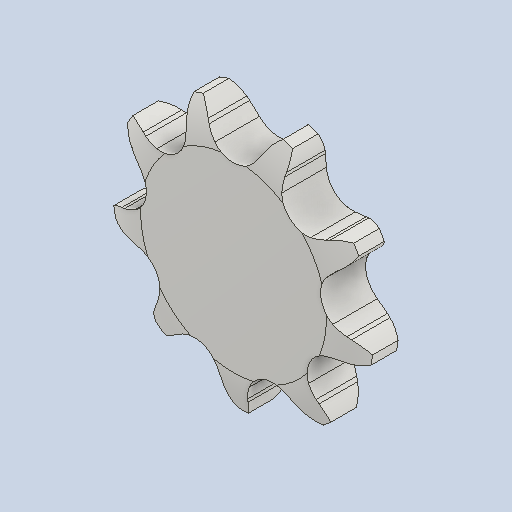
# Autodesk Inventor part: Rueda dentada de cadena de rodillos2
Saved by Autodesk Inventor 2022.1 (Build 261234000, 234)
## iProperties
CustomPartVersion: 1
Created: 2021-09-11
Part Number: Rueda dentada de cadena de rodillos2
Material: Steel
Document SubType Name: Modeling
Designer: seb_0
Density: 1 g/cm^3
Appearance: Steel
Author: seb_0
Autodesk Inventor part; units mm, degrees
ref_plane "YZ Plane" through (0, 0, 0) normal (1, 0, 0) x (0, 1, 0)
ref_plane "XZ Plane" through (0, 0, 0) normal (0, 1, 0) x (-1, 0, 0)
ref_plane "XY Plane" through (0, 0, 0) normal (0, 0, 1) x (1, 0, 0)
sketch "Perfil de diente teórico" plane through (0, 0, 0) normal (0, 0, 1) x (1, 0, 0)
  circle A0 centre (0, 0) radius 23.2077 construction
  line L0 (0, 0) -> (0, 23.2077) construction
  line L1 (0, 0) -> (14.9176, 17.7781) construction
  circle A1 centre (0, 0) radius 26.5706
  arc A2 (-3.8328, 19.7968) -> (3.8328, 19.7968) centre (0, 23.2077) ccw
  line L2 (0, 23.2077) -> (14.9176, 17.7781) construction
  line L3 (0, 23.2077) -> (6.0718, 28.6112) construction
  line L4 (6.0718, 28.6112) -> (-5.4235, 22.004) construction
  arc A3 (8.1227, 25.2986) -> (5.814, 22.6835) centre (13.3662, 18.3428) ccw
  arc A4 (-5.814, 22.6835) -> (-8.1227, 25.2986) centre (-13.3662, 18.3428) ccw
  line L5 (-13.3662, 18.3428) -> (-5.814, 22.6835) construction
  arc A5 (-5.4235, 22.004) -> (-3.8328, 19.7968) centre (6.0718, 28.6112) ccw
  line L6 (-5.4235, 22.004) -> (-5.814, 22.6835)
  arc A6 (3.8328, 19.7968) -> (5.4235, 22.004) centre (-6.0718, 28.6112) ccw
  line L7 (5.814, 22.6835) -> (5.4235, 22.004)
  line L8 (0, 0) -> (9.0877, 24.9682) construction
  point P0 (7.4588, 20.4929)
  dimension "d0" = 46.4154
  dimension "d2" = 40
  dimension "d3" = 5.1308
  dimension "d10" = 131.667
  dimension "d11" = 11.778
  dimension "d12" = 8.128
  dimension "d13" = 13.2588
  dimension "d14" = 14.224
  dimension "d23" = 4.7625
  constraints: 18 end point, 15 point on circle, 7 centre point, 3 coincident, 3 point on line, 3 symmetric about line, 3 tangent, 1 equal radius, 1 midpoint, 1 parallel, 1 vertical, 1 other
  measures "d0" diameter of A0
  measures "d2" angle of L1 L0
  measures "d3" radius of A2
  measures "d10" angle of L3 L0
  measures "d11" angle of L4 L3
  measures "d12" distance of L2.start L3.end
  measures "d13" distance of L3.end L4.end
  measures "d14" distance of A3.centre L0.end
  measures "d23" distance from line of L8.end L2
sketch "Perfil de diente" plane through (0, 0, 0) normal (0, 0, 1) x (1, 0, 0)
  arc A0 (-4.6501, 21.0393) -> (4.6501, 21.0393) centre (0, 23.2077) ccw
  arc A1 (7.8744, 25.377) -> (4.6501, 21.0393) centre (16.8048, 15.3715) ccw
  arc A2 (-4.6501, 21.0393) -> (-7.8744, 25.377) centre (-16.8048, 15.3715) ccw
  line L0 (0, 0) -> (0, 23.2077) construction
  line L1 (0, 23.2077) -> (4.6501, 21.0393) construction
  line L2 (0, 23.2077) -> (-4.6501, 21.0393) construction
  circle A3 centre (0, 0) radius 26.5706 projected
  dimension "d44" = 130
  dimension "d45" = 13.4112
  dimension "d46" = 5.1308
  constraints: 9 point on circle, 6 end point, 3 centre point, 2 tangent, 1 coincident, 1 equal radius, 1 vertical, 1 other
  measures "d44" angle of L2 L1
  measures "d45" radius of A1
  measures "d46" radius of A0
sketch "Perfil de sección" plane through (0, 0, 0) normal (1, 0, 0) x (0, 1, 0)
  line L0 (26.5706, 0) -> (-26.5706, 0) projected
  line L1 (9.7135, 4.5838) -> (-9.7135, 4.5838)
  line L2 (-9.7135, 4.5838) -> (-9.7135, -4.5838)
  line L3 (-9.7135, -4.5838) -> (9.7135, -4.5837)
  line L4 (9.7135, -4.5837) -> (9.7135, 4.5838)
  line L5 (9.7135, 4.5838) -> (26.5706, 4.5838) construction
  line L6 (26.5706, 4.5838) -> (26.5706, -4.5838) construction
  line L7 (26.5706, -4.5838) -> (9.7135, -4.5838) construction
  line L8 (9.7135, -4.5838) -> (9.7135, 4.5838)
  arc A0 (26.5706, 2.5994) -> (18.8852, 4.5838) centre (18.8852, -11.2913) ccw
  arc A1 (18.8852, -4.5838) -> (26.5706, -2.5994) centre (18.8852, 11.2913) ccw
  line L9 (18.8852, 4.5838) -> (0, 4.5838)
  line L10 (0, 4.5838) -> (0, -4.5838)
  line L11 (0, -4.5838) -> (18.8852, -4.5838)
  line L12 (0, 4.5838) -> (0, -4.5838)
  line L13 (26.5706, 2.5994) -> (26.5706, -2.5994)
  point P0 (0, 0)
  point P1 (0, 0)
  dimension "d30" = 9.1675
  dimension "d31" = 19.427
  dimension "d32" = 9.1675
  dimension "d33" = 1.9844
  dimension "d34" = 15.875
  dimension "d43" = 4.5838
  constraints: 26 end point, 7 midpoint, 5 perpendicular, 4 parallel, 4 point on circle, 3 point on line, 3 symmetric about line, 2 centre point, 2 horizontal, 2 tangent, 1 collinear, 1 other
  measures "d30" distance between parallel lines of L7 L5
  measures "d31" distance between parallel lines of L2 L4
  measures "d32" distance between parallel lines of L3 L1
  measures "d33" distance from line of L13.start L5
  measures "d34" radius of A0
  measures "d43" distance between parallel lines of L3 L0
revolve "Cubierta" add sketch "Perfil de sección" angle 360 about axis through (0, 0, 4.5838) along (0, 0, -1) contours L10 L3 L2 L0 | L0 L2 L1 L10
revolve "Ramal" add sketch "Perfil de sección" angle 360 about axis through (0, 0, 4.5838) along (0, 0, -1) contours L13 A1 L11 L4 L0 | L0 L4 L9 A0 L13 | L4 L3 L10 L0 | L0 L10 L1 L4
pattern_of_one "Patrón de ramal"
extrude "Diente teórico" cut sketch "Perfil de diente teórico" along normal through all both and the other way through all contours A3 L7 A6 A2 A5 L6 A4 A1 picked at (0.2056, 23.6569)
extrude "Diente" [suppressed]
pattern_circular "Patrón de diente" count 9 over 360 about axis through (0, 0, -10) along (0, 0, 1) of "Diente teórico"
ref_plane "Plano síncrono" through (0, 23.2077, 0) normal (1, 0, 0) x (0, 1, 0)
equation "\"d3\" = 0.5 * da_Dr + da_SC"
equation "\"d12\" = 0.8 * da_Dr"
equation "\"d13\" = 1.3 * da_Dr + da_SC"
equation "\"d14\" = 1.4 * da_Dr"
equation "\"d23\" = da_Ha"
equation "\"d44\" = da_Alfa"
equation "\"d45\" = da_Re"
equation "\"d46\" = da_Ri"
equation "\"d30\" = da_Bf"
equation "\"d31\" = da_Ds"
equation "\"d32\" = da_Bs"
equation "\"d33\" = da_Ba"
equation "\"d34\" = da_Rx"
equation "\"d40\" = da_pt"
equation "\"form_type\" = 0"
equation "\"da_p\" = 15.875"
equation "\"da_Dr\" = 10.16"
equation "\"da_SC\" = 0.0508"
equation "\"da_Ha\" = 4.7625"
equation "\"da_pt\" = 16.59"
equation "\"da_Bf\" = 9.1675"
equation "\"da_Ba\" = 1.98438"
equation "\"da_Rx\" = 15.875"
equation "\"da_Ra\" = 0.635"
equation "\"da_Bs\" = 9.1675"
equation "\"da_Ds\" = 19.427"
equation "\"da_Re\" = 13.4112"
equation "\"da_Ri\" = 5.1308"
equation "\"da_Alfa\" = 130deg"
body "Solid1"
